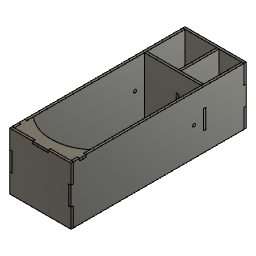
WeldingGearCubby (Autodesk Fusion 360 design; units mm, degrees)
Autodesk Fusion 360 part; units mm, degrees
note: some values were not read from the file. Set by a fixed rule: which face or edge a step refers to.
(part 1 of 2)
sketch "Sketch1" plane through (0, 0, 0) normal (0, 1, 0) x (1, 0, 0)
  line L0 (0, 0) -> (254, 0)
  line L1 (254, 0) -> (254, -304.8)
  line L2 (254, -304.8) -> (0, -304.8)
  line L3 (0, -304.8) -> (0, 0)
  line L4 (254, 0) -> (272.288, 0)
  line L5 (272.288, 0) -> (272.288, -304.8)
  line L6 (272.288, -304.8) -> (254, -304.8)
  line L7 (254, -304.8) -> (254, 0)
  line L8 (272.288, 0) -> (453.263, 0)
  line L9 (453.263, 0) -> (453.263, -304.8)
  line L10 (453.263, -304.8) -> (272.288, -304.8)
  line L11 (272.288, -304.8) -> (272.288, 0)
  line L12 (0, 0) -> (-18.288, 0) construction
  line L13 (-18.288, 0) -> (471.551, 0)
  line L14 (-18.288, 0) -> (0, 0)
  line L15 (0, 0) -> (0, -1364.488)
  line L16 (0, -1364.488) -> (-18.288, -1364.488)
  line L17 (-18.288, -1364.488) -> (-18.288, 0)
  line L18 (471.551, 0) -> (453.263, 0)
  line L19 (453.263, 0) -> (453.263, -1364.488)
  line L20 (453.263, -1364.488) -> (471.551, -1364.488)
  line L21 (471.551, -1364.488) -> (471.551, 0)
  line L22 (-18.288, -1364.488) -> (471.551, -1364.488)
  line L23 (471.551, -1364.488) -> (471.551, -1382.776)
  line L24 (471.551, -1382.776) -> (-18.288, -1382.776)
  line L25 (-18.288, -1382.776) -> (-18.288, -1364.488)
  line L26 (0, -304.8) -> (453.263, -304.8)
  line L27 (453.263, -304.8) -> (453.263, -323.088)
  line L28 (453.263, -323.088) -> (0, -323.088)
  line L29 (0, -323.088) -> (0, -304.8)
  line L30 (-18.288, 0) -> (-18.288, 18.288)
  line L31 (471.551, 0) -> (471.551, 18.288)
  line L32 (-18.288, 18.288) -> (471.551, 18.288)
  dimension "d2" = 254
  dimension "d3" = 304.8
  dimension "d4" = 18.288
  dimension "d5" = 304.8
  dimension "d6" = 180.975
  dimension "d7" = 304.8
  dimension "d8" = 18.288
  dimension "d9" = 489.839
  dimension "d10" = 1364.488
  dimension "d11" = 1364.488
  dimension "d12" = 489.839
  dimension "d13" = 18.288
  dimension "d14" = 453.263
  dimension "d15" = 18.288
  dimension "d30" = 18.288
  dimension "d31" = 18.288
  constraint horizontal L0
  constraint vertical L1
  constraint horizontal L2
  constraint vertical L3
  constraint coincident L0.start L3.end
  constraint horizontal L4
  constraint vertical L5
  constraint horizontal L6
  constraint vertical L7
  constraint horizontal L8
  constraint vertical L9
  constraint horizontal L10
  constraint vertical L11
  constraint perpendicular L3 L12
  constraint horizontal L13
  constraint horizontal L14
  constraint vertical L15
  constraint horizontal L16
  constraint vertical L17
  constraint horizontal L18
  constraint vertical L19
  constraint horizontal L20
  constraint vertical L21
  constraint horizontal L22
  constraint vertical L23
  constraint horizontal L24
  constraint vertical L25
  constraint horizontal L26
  constraint vertical L27
  constraint horizontal L28
  constraint vertical L29
  constraint perpendicular L13 L30
  constraint perpendicular L18 L31
  measures "d2" distance of L0.start L0.end
  measures "d3" distance of L0.start L2.end
  measures "d4" distance of L0.end L4.end
  measures "d5" distance of L0.end L1.end
  measures "d6" distance of L4.end L8.end
  measures "d7" distance of L4.end L5.end
  measures "d8" distance of L0.start L12.end
  measures "d9" distance of L12.end L13.end
  measures "d10" distance of L12.end L16.end
  measures "d11" distance of L13.end L20.end
  measures "d12" distance of L16.end L20.end
  measures "d13" distance of L16.end L24.end
  measures "d14" distance of L2.end L9.end
  measures "d15" distance of L2.end L28.end
  measures "d30" distance of L12.end L30.end
  measures "d31" distance of L13.end L31.end
extrude "Extrude1" add sketch "Sketch1" against normal blind 457.2 contours L0 L4 L8 L13 L14 L18 L30 L31 L32 makes body 1
copy_body "Body->Comp1" bodies 1 removing the originals makes body 2 in component "Top"
extrude "Extrude1'" add sketch "Sketch1" against normal blind 457.2 separate body contours L3 L13 L14 L15 L16 L17 L22 L29 makes body 3 in component "RightSide"
extrude "Extrude1''" add sketch "Sketch1" against normal blind 457.2 separate body contours L9 L13 L18 L19 L20 L21 L22 L27 makes body 4 in component "LeftSide"
extrude "Extrude1'''" add sketch "Sketch1" against normal blind 457.2 separate body contours L1 L4 L5 L6 L7 L11 L13 L26 makes body 5 in component "Divider"
extrude "Extrude1''''" add sketch "Sketch1" against normal blind 457.2 separate body contours L2 L6 L10 L15 L19 L26 L27 L28 L29 makes body 6 in component "Shelf"
extrude "Extrude1'''''" add sketch "Sketch1" against normal blind 457.2 separate body contours L16 L20 L22 L23 L24 L25 makes body 7 in component "Bottom"
extrude "Extrude1''''''" add sketch "Sketch1" along normal blind 18.288 separate body makes body 8 in component "Back"
sketch "Sketch2" plane through (0, 0, -18.288) normal (0, 0, -1) x (-1, 0, 0)
  line L0 (18.288, 0) -> (-471.551, 0)
  line L1 (-471.551, 0) -> (-471.551, -457.2)
  line L2 (-471.551, -457.2) -> (18.288, -457.2)
  line L3 (18.288, -457.2) -> (18.288, 0)
  line L4 (-150.4315, -18.288) -> (-302.8315, -18.288)
  line L5 (-302.8315, -18.288) -> (-302.8315, 18.288)
  line L6 (-302.8315, 18.288) -> (-150.4315, 18.288)
  line L7 (-150.4315, 18.288) -> (-150.4315, -18.288)
  line L8 (-150.4315, -18.288) -> (-302.8315, 18.288) construction
  line L9 (-302.8315, -18.288) -> (-150.4315, 18.288) construction
  line L10 (-453.263, -304.8) -> (-489.839, -304.8)
  line L11 (-489.839, -304.8) -> (-489.839, -152.4)
  line L12 (-489.839, -152.4) -> (-453.263, -152.4)
  line L13 (-453.263, -152.4) -> (-453.263, -304.8)
  line L14 (-453.263, -304.8) -> (-489.839, -152.4) construction
  line L15 (-489.839, -304.8) -> (-453.263, -152.4) construction
  line L16 (36.576, -304.8) -> (0, -304.8)
  line L17 (0, -304.8) -> (0, -152.4)
  line L18 (0, -152.4) -> (36.576, -152.4)
  line L19 (36.576, -152.4) -> (36.576, -304.8)
  line L20 (36.576, -304.8) -> (0, -152.4) construction
  line L21 (0, -304.8) -> (36.576, -152.4) construction
  point P0 (-226.6315, 0)
  point P1 (-471.551, -228.6)
  point P2 (18.288, -228.6)
  dimension "d32" = 152.4
  dimension "d33" = 36.576
  dimension "d34" = 36.576
  dimension "d35" = 152.4
  dimension "d36" = 36.576
  dimension "d37" = 152.4
  constraint horizontal L4
  constraint perpendicular L4 L5
  constraint parallel L4 L6
  constraint parallel L5 L7
  constraint coincident L8 P0
  constraint coincident L9 P0
  constraint midpoint L0 P0
  constraint horizontal L10
  constraint perpendicular L10 L11
  constraint parallel L10 L12
  constraint parallel L11 L13
  constraint coincident L14 P1
  constraint coincident L15 P1
  constraint midpoint L1 P1
  constraint horizontal L16
  constraint perpendicular L16 L17
  constraint parallel L16 L18
  constraint parallel L17 L19
  constraint coincident L20 P2
  constraint coincident L21 P2
  constraint midpoint L3 P2
  measures "d32" distance of L5.end L6.end
  measures "d33" distance of L4.end L5.end
  measures "d34" distance of L11.end L12.end
  measures "d35" distance of L10.end L11.end
  measures "d36" distance of L17.end L18.end
  measures "d37" distance of L16.end L17.end
extrude "Extrude1'''''''" add sketch "Sketch2" against normal up to surface (18.288 mm away) contours L0 L5 L6 L7 bodies 2 in component "Top"
extrude "Extrude2" cut sketch "Sketch2" against normal up to surface (18.288 mm away) contours L3 L16 L17 L18 | L1 L10 L12 L13 bodies 2 in component "Top"
sketch "Sketch3" plane through (0, 0, 1382.776) normal (0, 0, 1) x (1, 0, 0)
  line L0 (471.551, 0) -> (-18.288, 0)
  line L1 (-18.288, 0) -> (-18.288, -457.2)
  line L2 (-18.288, -457.2) -> (471.551, -457.2)
  line L3 (471.551, -457.2) -> (471.551, 0)
  line L4 (489.839, -304.8) -> (453.263, -304.8)
  line L5 (453.263, -304.8) -> (453.263, -152.4)
  line L6 (453.263, -152.4) -> (489.839, -152.4)
  line L7 (489.839, -152.4) -> (489.839, -304.8)
  line L8 (489.839, -304.8) -> (453.263, -152.4) construction
  line L9 (453.263, -304.8) -> (489.839, -152.4) construction
  line L10 (0, -304.8) -> (-36.576, -304.8)
  line L11 (-36.576, -304.8) -> (-36.576, -152.4)
  line L12 (-36.576, -152.4) -> (0, -152.4)
  line L13 (0, -152.4) -> (0, -304.8)
  line L14 (0, -304.8) -> (-36.576, -152.4) construction
  line L15 (-36.576, -304.8) -> (0, -152.4) construction
  line L16 (312.4324, 18.288) -> (140.8306, 18.288)
  line L17 (140.8306, 18.288) -> (140.8306, -18.288)
  line L18 (140.8306, -18.288) -> (312.4324, -18.288)
  line L19 (312.4324, -18.288) -> (312.4324, 18.288)
  line L20 (312.4324, 18.288) -> (140.8306, -18.288) construction
  line L21 (140.8306, 18.288) -> (312.4324, -18.288) construction
  point P0 (471.551, -228.6)
  point P1 (-18.288, -228.6)
  point P2 (226.6315, 0)
  dimension "d42" = 36.576
  dimension "d43" = 152.4
  dimension "d44" = 36.576
  dimension "d45" = 152.4
  dimension "d46" = 36.576
  constraint horizontal L4
  constraint perpendicular L4 L5
  constraint parallel L4 L6
  constraint parallel L5 L7
  constraint coincident L8 P0
  constraint coincident L9 P0
  constraint midpoint L3 P0
  constraint horizontal L10
  constraint perpendicular L10 L11
  constraint parallel L10 L12
  constraint parallel L11 L13
  constraint coincident L14 P1
  constraint coincident L15 P1
  constraint midpoint L1 P1
  constraint horizontal L16
  constraint perpendicular L16 L17
  constraint parallel L16 L18
  constraint parallel L17 L19
  constraint coincident L20 P2
  constraint coincident L21 P2
  constraint midpoint L0 P2
  measures "d42" distance of L5.end L6.end
  measures "d43" distance of L4.end L5.end
  measures "d44" distance of L11.end L12.end
  measures "d45" distance of L10.end L11.end
  measures "d46" distance of L16.end L17.end
extrude "Extrude2'" add sketch "Sketch3" against normal up to surface (18.288 mm away) contours L0 L16 L17 L19 bodies 7 in component "Bottom"
extrude "Extrude3" cut sketch "Sketch3" against normal up to surface (18.288 mm away) contours L3 L4 L5 L6 | L1 L10 L12 L13 bodies 7 in component "Bottom"
sketch "Sketch4" plane through (0, 0, -18.288) normal (0, 0, -1) x (-1, 0, 0)
  line L0 (-453.263, -304.8) -> (-471.551, -304.8)
  line L1 (-471.551, -304.8) -> (-471.551, -457.2)
  line L2 (-471.551, -457.2) -> (18.288, -457.2)
  line L3 (18.288, -457.2) -> (18.288, -304.8)
  line L4 (18.288, -304.8) -> (0, -304.8)
  line L5 (0, -304.8) -> (0, -152.4)
  line L6 (0, -152.4) -> (18.288, -152.4)
  line L7 (18.288, -152.4) -> (18.288, 0)
  line L8 (18.288, 0) -> (-150.4315, 0)
  line L9 (-150.4315, 0) -> (-150.4315, 18.288)
  line L10 (-150.4315, 18.288) -> (-302.8315, 18.288)
  line L11 (-302.8315, 18.288) -> (-302.8315, 0)
  line L12 (-302.8315, 0) -> (-471.551, 0)
  line L13 (-471.551, 0) -> (-471.551, -152.4)
  line L14 (-471.551, -152.4) -> (-453.263, -152.4)
  line L15 (-453.263, -152.4) -> (-453.263, -304.8)
  line L16 (-453.263, -228.6) -> (-263.144, -228.6) construction
  line L17 (-254, -304.8) -> (-272.288, -304.8)
  line L18 (-272.288, -304.8) -> (-272.288, -152.4)
  line L19 (-272.288, -152.4) -> (-254, -152.4)
  line L20 (-254, -152.4) -> (-254, -304.8)
  line L21 (-254, -304.8) -> (-272.288, -152.4) construction
  line L22 (-272.288, -304.8) -> (-254, -152.4) construction
  point P0 (-263.144, -228.6)
  dimension "d51" = 190.119
  dimension "d52" = 18.288
  dimension "d53" = 152.4
  constraint midpoint L15 L16.start
  constraint perpendicular L15 L16
  constraint horizontal L17
  constraint perpendicular L17 L18
  constraint parallel L17 L19
  constraint parallel L18 L20
  constraint coincident L21 P0
  constraint coincident L22 P0
  constraint coincident P0 L16.end
  measures "d51" distance of L16.start P0
  measures "d52" distance of L18.end L19.end
  measures "d53" distance of L17.end L18.end
extrude "Extrude3'" cut sketch "Sketch4" against normal blind 18.288 contours L17 L18 L19 L20 bodies 2 in component "Top"
sketch "Sketch5" plane through (0, 0, 304.8) normal (0, 0, -1) x (-1, 0, 0)
  line L0 (0, 0) -> (-453.263, 0)
  line L1 (-453.263, 0) -> (-453.263, -457.2)
  line L2 (-453.263, -457.2) -> (0, -457.2)
  line L3 (0, -457.2) -> (0, 0)
  line L4 (-150.4315, 18.288) -> (-302.8315, 18.288)
  line L5 (-302.8315, 18.288) -> (-302.8315, -18.288)
  line L6 (-302.8315, -18.288) -> (-150.4315, -18.288)
  line L7 (-150.4315, -18.288) -> (-150.4315, 18.288)
  line L8 (-150.4315, 18.288) -> (-302.8315, -18.288) construction
  line L9 (-302.8315, 18.288) -> (-150.4315, -18.288) construction
  line L10 (18.288, -304.8) -> (-18.288, -304.8)
  line L11 (-18.288, -304.8) -> (-18.288, -152.4)
  line L12 (-18.288, -152.4) -> (18.288, -152.4)
  line L13 (18.288, -152.4) -> (18.288, -304.8)
  line L14 (18.288, -304.8) -> (-18.288, -152.4) construction
  line L15 (-18.288, -304.8) -> (18.288, -152.4) construction
  line L16 (-471.551, -304.8) -> (-434.975, -304.8)
  line L17 (-434.975, -304.8) -> (-434.975, -152.4)
  line L18 (-434.975, -152.4) -> (-471.551, -152.4)
  line L19 (-471.551, -152.4) -> (-471.551, -304.8)
  line L20 (-471.551, -304.8) -> (-434.975, -152.4) construction
  line L21 (-434.975, -304.8) -> (-471.551, -152.4) construction
  point P0 (-226.6315, 0)
  point P1 (0, -228.6)
  point P2 (-453.263, -228.6)
  dimension "d56" = 152.4
  dimension "d57" = 36.576
  dimension "d58" = 36.576
  dimension "d59" = 36.576
  constraint horizontal L4
  constraint perpendicular L4 L5
  constraint parallel L4 L6
  constraint parallel L5 L7
  constraint coincident L8 P0
  constraint coincident L9 P0
  constraint midpoint L0 P0
  constraint horizontal L10
  constraint perpendicular L10 L11
  constraint parallel L10 L12
  constraint parallel L11 L13
  constraint coincident L14 P1
  constraint coincident L15 P1
  constraint midpoint L3 P1
  constraint horizontal L16
  constraint perpendicular L16 L17
  constraint parallel L16 L18
  constraint parallel L17 L19
  constraint coincident L20 P2
  constraint coincident L21 P2
  constraint midpoint L1 P2
  measures "d56" distance of L5.end L6.end
  measures "d57" distance of L4.end L5.end
  measures "d58" distance of L11.end L12.end
  measures "d59" distance of L17.end L18.end
extrude "Extrude2''" add sketch "Sketch5" against normal up to surface (18.288 mm away) contours L0 L4 L5 L7 | L3 L10 L12 L13 | L1 L16 L18 L19 bodies 6 in component "Shelf"
sketch "Sketch6" plane through (0, 0, 304.8) normal (0, 0, -1) x (-1, 0, 0)
  line L0 (0, 0) -> (-150.4315, 0)
  line L1 (-150.4315, 0) -> (-150.4315, 18.288)
  line L2 (-150.4315, 18.288) -> (-302.8315, 18.288)
  line L3 (-302.8315, 18.288) -> (-302.8315, 0)
  line L4 (-302.8315, 0) -> (-453.263, 0)
  line L5 (-453.263, 0) -> (-453.263, -152.4)
  line L6 (-453.263, -152.4) -> (-471.551, -152.4)
  line L7 (-471.551, -152.4) -> (-471.551, -304.8)
  line L8 (-471.551, -304.8) -> (-453.263, -304.8)
  line L9 (-453.263, -304.8) -> (-453.263, -457.2)
  line L10 (-453.263, -457.2) -> (0, -457.2)
  line L11 (0, -457.2) -> (0, -304.8)
  line L12 (0, -304.8) -> (18.288, -304.8)
  line L13 (18.288, -304.8) -> (18.288, -152.4)
  line L14 (18.288, -152.4) -> (0, -152.4)
  line L15 (0, -152.4) -> (0, 0)
  line L16 (-471.551, -228.6) -> (-263.144, -228.6) construction
  line L17 (-254, -304.8) -> (-272.288, -304.8)
  line L18 (-272.288, -304.8) -> (-272.288, -152.4)
  line L19 (-272.288, -152.4) -> (-254, -152.4)
  line L20 (-254, -152.4) -> (-254, -304.8)
  line L21 (-254, -304.8) -> (-272.288, -152.4) construction
  line L22 (-272.288, -304.8) -> (-254, -152.4) construction
  point P0 (-263.144, -228.6)
  dimension "d62" = 208.407
  dimension "d63" = 18.288
  dimension "d64" = 152.4
  constraint midpoint L7 L16.start
  constraint perpendicular L7 L16
  constraint horizontal L17
  constraint perpendicular L17 L18
  constraint parallel L17 L19
  constraint parallel L18 L20
  constraint coincident L21 P0
  constraint coincident L22 P0
  constraint coincident P0 L16.end
  measures "d62" distance of L16.start P0
  measures "d63" distance of L18.end L19.end
  measures "d64" distance of L17.end L18.end
extrude "Extrude3''" cut sketch "Sketch6" against normal up to surface (18.288 mm away) contours L17 L18 L19 L20 bodies 6 in component "Shelf"
sketch "Sketch7" plane through (471.551, 0, 0) normal (1, 0, 0) x (0, 0, -1)
  line L0 (0, 0) -> (-1364.488, 0)
  line L1 (-1364.488, 0) -> (-1364.488, -457.2)
  line L2 (-1364.488, -457.2) -> (0, -457.2)
  line L3 (0, -457.2) -> (0, 0)
  line L4 (18.288, -304.8) -> (-18.288, -304.8)
  line L5 (-18.288, -304.8) -> (-18.288, -152.4)
  line L6 (-18.288, -152.4) -> (18.288, -152.4)
  line L7 (18.288, -152.4) -> (18.288, -304.8)
  line L8 (18.288, -304.8) -> (-18.288, -152.4) construction
  line L9 (-18.288, -304.8) -> (18.288, -152.4) construction
  line L10 (0, -228.6) -> (-313.944, -228.6) construction
  line L11 (-304.8, -304.8) -> (-323.088, -304.8)
  line L12 (-323.088, -304.8) -> (-323.088, -152.4)
  line L13 (-323.088, -152.4) -> (-304.8, -152.4)
  line L14 (-304.8, -152.4) -> (-304.8, -304.8)
  line L15 (-304.8, -304.8) -> (-323.088, -152.4) construction
  line L16 (-323.088, -304.8) -> (-304.8, -152.4) construction
  line L17 (-1382.776, -304.8) -> (-1346.2, -304.8)
  line L18 (-1346.2, -304.8) -> (-1346.2, -152.4)
  line L19 (-1346.2, -152.4) -> (-1382.776, -152.4)
  line L20 (-1382.776, -152.4) -> (-1382.776, -304.8)
  line L21 (-1382.776, -304.8) -> (-1346.2, -152.4) construction
  line L22 (-1346.2, -304.8) -> (-1382.776, -152.4) construction
  point P0 (0, -228.6)
  point P1 (-313.944, -228.6)
  point P2 (-1364.488, -228.6)
  dimension "d67" = 36.576
  dimension "d68" = 313.944
  dimension "d69" = 18.288
  dimension "d70" = 152.4
  dimension "d71" = 36.576
  dimension "d72" = 152.4
  constraint horizontal L4
  constraint perpendicular L4 L5
  constraint parallel L4 L6
  constraint parallel L5 L7
  constraint coincident L8 P0
  constraint coincident L9 P0
  constraint midpoint L3 P0
  constraint coincident P0 L10.start
  constraint perpendicular L5 L10
  constraint horizontal L11
  constraint perpendicular L11 L12
  constraint parallel L11 L13
  constraint parallel L12 L14
  constraint coincident L15 P1
  constraint coincident L16 P1
  constraint coincident P1 L10.end
  constraint horizontal L17
  constraint perpendicular L17 L18
  constraint parallel L17 L19
  constraint parallel L18 L20
  constraint coincident L21 P2
  constraint coincident L22 P2
  constraint midpoint L1 P2
  measures "d67" distance of L5.end L6.end
  measures "d68" distance of P0 P1
  measures "d69" distance of L12.end L13.end
  measures "d70" distance of L11.end L12.end
  measures "d71" distance of L18.end L19.end
  measures "d72" distance of L17.end L18.end
extrude "Extrude2'''" add sketch "Sketch7" against normal up to surface (18.288 mm away) contours L3 L4 L6 L7 | L1 L17 L19 L20 bodies 4 in component "LeftSide"
extrude "Extrude3'''" cut sketch "Sketch7" against normal up to surface (18.288 mm away) contours L11 L12 L13 L14 bodies 4 in component "LeftSide"
sketch "Sketch8" plane through (-18.288, 0, 0) normal (-1, 0, 0) x (0, 0, 1)
  line L0 (1364.488, 0) -> (0, 0)
  line L1 (0, 0) -> (0, -457.2)
  line L2 (0, -457.2) -> (1364.488, -457.2)
  line L3 (1364.488, -457.2) -> (1364.488, 0)
  line L4 (18.288, -304.8) -> (-18.288, -304.8)
  line L5 (-18.288, -304.8) -> (-18.288, -152.4)
  line L6 (-18.288, -152.4) -> (18.288, -152.4)
  line L7 (18.288, -152.4) -> (18.288, -304.8)
  line L8 (18.288, -304.8) -> (-18.288, -152.4) construction
  line L9 (-18.288, -304.8) -> (18.288, -152.4) construction
  line L10 (1382.776, -304.8) -> (1346.2, -304.8)
  line L11 (1346.2, -304.8) -> (1346.2, -152.4)
  line L12 (1346.2, -152.4) -> (1382.776, -152.4)
  line L13 (1382.776, -152.4) -> (1382.776, -304.8)
  line L14 (1382.776, -304.8) -> (1346.2, -152.4) construction
  line L15 (1346.2, -304.8) -> (1382.776, -152.4) construction
  line L16 (0, -228.6) -> (313.944, -228.6) construction
  line L17 (323.088, -304.8) -> (304.8, -304.8)
  line L18 (304.8, -304.8) -> (304.8, -152.4)
  line L19 (304.8, -152.4) -> (323.088, -152.4)
  line L20 (323.088, -152.4) -> (323.088, -304.8)
  line L21 (323.088, -304.8) -> (304.8, -152.4) construction
  line L22 (304.8, -304.8) -> (323.088, -152.4) construction
  point P0 (0, -228.6)
  point P1 (1364.488, -228.6)
  point P2 (313.944, -228.6)
  dimension "d77" = 36.576
  dimension "d78" = 152.4
  dimension "d79" = 36.576
  dimension "d80" = 152.4
  dimension "d81" = 313.944
  dimension "d82" = 18.288
  dimension "d83" = 152.4
  constraint horizontal L4
  constraint perpendicular L4 L5
  constraint parallel L4 L6
  constraint parallel L5 L7
  constraint coincident L8 P0
  constraint coincident L9 P0
  constraint midpoint L1 P0
  constraint horizontal L10
  constraint perpendicular L10 L11
  constraint parallel L10 L12
  constraint parallel L11 L13
  constraint coincident L14 P1
  constraint coincident L15 P1
  constraint midpoint L3 P1
  constraint coincident P0 L16.start
  constraint perpendicular L7 L16
  constraint horizontal L17
  constraint perpendicular L17 L18
  constraint parallel L17 L19
  constraint parallel L18 L20
  constraint coincident L21 P2
  constraint coincident L22 P2
  constraint coincident P2 L16.end
  measures "d77" distance of L5.end L6.end
  measures "d78" distance of L4.end L5.end
  measures "d79" distance of L11.end L12.end
  measures "d80" distance of L10.end L11.end
  measures "d81" distance of P0 P2
  measures "d82" distance of L18.end L19.end
  measures "d83" distance of L17.end L18.end
extrude "Extrude2''''" add sketch "Sketch8" against normal up to surface (18.288 mm away) contours L3 L10 L12 L13 | L1 L4 L5 L6 bodies 3 in component "RightSide"
extrude "Extrude3''''" cut sketch "Sketch8" against normal up to surface (18.288 mm away) contours L17 L18 L19 L20 bodies 3 in component "RightSide"
sketch "Sketch9" plane through (272.288, 0, 0) normal (1, 0, 0) x (0, 0, -1)
  line L0 (0, 0) -> (-304.8, 0)
  line L1 (-304.8, 0) -> (-304.8, -457.2)
  line L2 (-304.8, -457.2) -> (0, -457.2)
  line L3 (0, -457.2) -> (0, 0)
  line L4 (18.288, -304.8) -> (-18.288, -304.8)
  line L5 (-18.288, -304.8) -> (-18.288, -152.4)
  line L6 (-18.288, -152.4) -> (18.288, -152.4)
  line L7 (18.288, -152.4) -> (18.288, -304.8)
  line L8 (18.288, -304.8) -> (-18.288, -152.4) construction
  line L9 (-18.288, -304.8) -> (18.288, -152.4) construction
  line L10 (-286.512, -304.8) -> (-323.088, -304.8)
  line L11 (-323.088, -304.8) -> (-323.088, -152.4)
  line L12 (-323.088, -152.4) -> (-286.512, -152.4)
  line L13 (-286.512, -152.4) -> (-286.512, -304.8)
  line L14 (-286.512, -304.8) -> (-323.088, -152.4) construction
  line L15 (-323.088, -304.8) -> (-286.512, -152.4) construction
  point P0 (0, -228.6)
  point P1 (-304.8, -228.6)
  dimension "d88" = 36.576
  dimension "d89" = 152.4
  dimension "d90" = 36.576
  constraint horizontal L4
  constraint perpendicular L4 L5
  constraint parallel L4 L6
  constraint parallel L5 L7
  constraint coincident L8 P0
  constraint coincident L9 P0
  constraint midpoint L3 P0
  constraint horizontal L10
  constraint perpendicular L10 L11
  constraint parallel L10 L12
  constraint parallel L11 L13
  constraint coincident L14 P1
  constraint coincident L15 P1
  constraint midpoint L1 P1
  measures "d88" distance of L5.end L6.end
  measures "d89" distance of L4.end L5.end
  measures "d90" distance of L11.end L12.end
extrude "Extrude2'''''" add sketch "Sketch9" against normal up to surface (18.288 mm away) contours L3 L4 L6 L7 | L1 L10 L11 L12 bodies 5 in component "Divider"
sketch "Sketch10" plane through (0, 18.288, 0) normal (0, 1, 0) x (-1, 0, 0)
  line L0 (18.288, -18.288) -> (18.288, 1382.776)
  line L1 (18.288, 1382.776) -> (-471.551, 1382.776)
  line L2 (-471.551, 1382.776) -> (-471.551, -18.288)
  line L3 (-471.551, -18.288) -> (18.288, -18.288)
  line L4 (-226.6315, -18.288) -> (-226.6315, 313.944) construction
  line L5 (-302.8315, 323.088) -> (-150.4315, 323.088)
  line L6 (-150.4315, 323.088) -> (-150.4315, 304.8)
  line L7 (-150.4315, 304.8) -> (-302.8315, 304.8)
  line L8 (-302.8315, 304.8) -> (-302.8315, 323.088)
  line L9 (-302.8315, 323.088) -> (-150.4315, 304.8) construction
  line L10 (-150.4315, 323.088) -> (-302.8315, 304.8) construction
  line L11 (-302.8315, 0) -> (-150.4315, 0)
  line L12 (-150.4315, 0) -> (-150.4315, -36.576)
  line L13 (-150.4315, -36.576) -> (-302.8315, -36.576)
  line L14 (-302.8315, -36.576) -> (-302.8315, 0)
  line L15 (-302.8315, 0) -> (-150.4315, -36.576) construction
  line L16 (-150.4315, 0) -> (-302.8315, -36.576) construction
  line L17 (-302.8315, 1401.064) -> (-150.4315, 1401.064)
  line L18 (-150.4315, 1401.064) -> (-150.4315, 1364.488)
  line L19 (-150.4315, 1364.488) -> (-302.8315, 1364.488)
  line L20 (-302.8315, 1364.488) -> (-302.8315, 1401.064)
  line L21 (-302.8315, 1401.064) -> (-150.4315, 1364.488) construction
  line L22 (-150.4315, 1401.064) -> (-302.8315, 1364.488) construction
  line L23 (-489.839, 758.444) -> (-453.263, 758.444)
  line L24 (-453.263, 758.444) -> (-453.263, 606.044)
  line L25 (-453.263, 606.044) -> (-489.839, 606.044)
  line L26 (-489.839, 606.044) -> (-489.839, 758.444)
  line L27 (-489.839, 758.444) -> (-453.263, 606.044) construction
  line L28 (-453.263, 758.444) -> (-489.839, 606.044) construction
  line L29 (0, 758.444) -> (36.576, 758.444)
  line L30 (36.576, 758.444) -> (36.576, 606.044)
  line L31 (36.576, 606.044) -> (0, 606.044)
  line L32 (0, 606.044) -> (0, 758.444)
  line L33 (0, 758.444) -> (36.576, 606.044) construction
  line L34 (36.576, 758.444) -> (0, 606.044) construction
  point P0 (-226.6315, 313.944)
  point P1 (-226.6315, -18.288)
  point P2 (-226.6315, 1382.776)
  point P3 (-471.551, 682.244)
  point P4 (18.288, 682.244)
  dimension "d93" = 332.232
  dimension "d94" = 152.4
  dimension "d95" = 18.288
  dimension "d96" = 152.4
  dimension "d97" = 36.576
  dimension "d98" = 152.4
  dimension "d99" = 36.576
  dimension "d100" = 36.576
  dimension "d101" = 152.4
  dimension "d102" = 36.576
  dimension "d103" = 152.4
  constraint midpoint L3 P1
  constraint perpendicular L3 L4
  constraint horizontal L5
  constraint perpendicular L5 L6
  constraint parallel L5 L7
  constraint parallel L6 L8
  constraint coincident L9 P0
  constraint coincident L10 P0
  constraint coincident P0 L4.end
  constraint horizontal L11
  constraint perpendicular L11 L12
  constraint parallel L11 L13
  constraint parallel L12 L14
  constraint coincident L15 P1
  constraint coincident L16 P1
  constraint coincident P1 L4.start
  constraint horizontal L17
  constraint perpendicular L17 L18
  constraint parallel L17 L19
  constraint parallel L18 L20
  constraint coincident L21 P2
  constraint coincident L22 P2
  constraint midpoint L1 P2
  constraint horizontal L23
  constraint perpendicular L23 L24
  constraint parallel L23 L25
  constraint parallel L24 L26
  constraint coincident L27 P3
  constraint coincident L28 P3
  constraint midpoint L2 P3
  constraint horizontal L29
  constraint perpendicular L29 L30
  constraint parallel L29 L31
  constraint parallel L30 L32
  constraint coincident L33 P4
  constraint coincident L34 P4
  constraint midpoint L0 P4
  measures "d93" distance of P1 P0
  measures "d94" distance of L6.end L7.end
  measures "d95" distance of L5.end L6.end
  measures "d96" distance of L12.end L13.end
  measures "d97" distance of L11.end L12.end
  measures "d98" distance of L18.end L19.end
  measures "d99" distance of L17.end L18.end
  measures "d100" distance of L24.end L25.end
  measures "d101" distance of L23.end L24.end
  measures "d102" distance of L30.end L31.end
  measures "d103" distance of L29.end L30.end
extrude "Extrude2''''''" cut sketch "Sketch10" against normal up to surface (18.288 mm away) contours L0 L29 L31 L32 | L3 L11 L12 L14 | L1 L18 L19 L20 | L2 L23 L24 L25 | L5 L6 L7 L8 bodies 8 in component "Back"
sketch "Sketch11" plane through (471.551, 0, 0) normal (1, 0, 0) x (0, 0, -1)
  line L0 (-304.8, -152.4) -> (-304.8, -304.8)
  line L1 (-304.8, -304.8) -> (-323.088, -304.8)
  line L2 (-323.088, -304.8) -> (-323.088, -152.4)
  line L3 (-323.088, -152.4) -> (-304.8, -152.4)
  line L4 (0, 0) -> (-1364.488, 0)
  line L5 (-1364.488, 0) -> (-1364.488, -152.4)
  line L6 (-1364.488, -152.4) -> (-1382.776, -152.4)
  line L7 (-1382.776, -152.4) -> (-1382.776, -304.8)
  line L8 (-1382.776, -304.8) -> (-1364.488, -304.8)
  line L9 (-1364.488, -304.8) -> (-1364.488, -457.2)
  line L10 (-1364.488, -457.2) -> (0, -457.2)
  line L11 (0, -457.2) -> (0, -304.8)
  line L12 (0, -304.8) -> (18.288, -304.8)
  line L13 (18.288, -304.8) -> (18.288, -152.4)
  line L14 (18.288, -152.4) -> (0, -152.4)
  line L15 (0, -152.4) -> (0, 0)
  line L16 (-606.044, 18.288) -> (-758.444, 18.288)
  line L17 (-758.444, 18.288) -> (-758.444, -18.288)
  line L18 (-758.444, -18.288) -> (-606.044, -18.288)
  line L19 (-606.044, -18.288) -> (-606.044, 18.288)
  line L20 (-606.044, 18.288) -> (-758.444, -18.288) construction
  line L21 (-758.444, 18.288) -> (-606.044, -18.288) construction
  point P0 (-682.244, 0)
  dimension "d106" = 152.4
  dimension "d107" = 36.576
  constraint horizontal L16
  constraint perpendicular L16 L17
  constraint parallel L16 L18
  constraint parallel L17 L19
  constraint coincident L20 P0
  constraint coincident L21 P0
  constraint midpoint L4 P0
  measures "d106" distance of L17.end L18.end
  measures "d107" distance of L16.end L17.end
extrude "Extrude4" add sketch "Sketch11" against normal up to surface (18.288 mm away) contours L4 L16 L17 L19 bodies 4 in component "LeftSide"
sketch "Sketch12" plane through (-18.288, 0, 0) normal (-1, 0, 0) x (0, 0, 1)
  line L0 (323.088, -152.4) -> (323.088, -304.8)
  line L1 (323.088, -304.8) -> (304.8, -304.8)
  line L2 (304.8, -304.8) -> (304.8, -152.4)
  line L3 (304.8, -152.4) -> (323.088, -152.4)
  line L4 (1364.488, 0) -> (0, 0)
  line L5 (0, 0) -> (0, -152.4)
  line L6 (0, -152.4) -> (-18.288, -152.4)
  line L7 (-18.288, -152.4) -> (-18.288, -304.8)
  line L8 (-18.288, -304.8) -> (0, -304.8)
  line L9 (0, -304.8) -> (0, -457.2)
  line L10 (0, -457.2) -> (1364.488, -457.2)
  line L11 (1364.488, -457.2) -> (1364.488, -304.8)
  line L12 (1364.488, -304.8) -> (1382.776, -304.8)
  line L13 (1382.776, -304.8) -> (1382.776, -152.4)
  line L14 (1382.776, -152.4) -> (1364.488, -152.4)
  line L15 (1364.488, -152.4) -> (1364.488, 0)
  line L16 (758.444, 18.288) -> (606.044, 18.288)
  line L17 (606.044, 18.288) -> (606.044, -18.288)
  line L18 (606.044, -18.288) -> (758.444, -18.288)
  line L19 (758.444, -18.288) -> (758.444, 18.288)
  line L20 (758.444, 18.288) -> (606.044, -18.288) construction
  line L21 (606.044, 18.288) -> (758.444, -18.288) construction
  point P0 (682.244, 0)
  dimension "d110" = 152.4
  dimension "d111" = 36.576
  constraint horizontal L16
  constraint perpendicular L16 L17
  constraint parallel L16 L18
  constraint parallel L17 L19
  constraint coincident L20 P0
  constraint coincident L21 P0
  constraint midpoint L4 P0
  measures "d110" distance of L17.end L18.end
  measures "d111" distance of L16.end L17.end
extrude "Extrude4'" add sketch "Sketch12" against normal up to surface (18.288 mm away) contours L4 L16 L17 L19 bodies 3 in component "RightSide"
sketch "Sketch13" plane through (471.551, 0, 0) normal (1, 0, 0) x (0, 0, -1)
  line L0 (-304.8, -152.4) -> (-304.8, -304.8)
  line L1 (-304.8, -304.8) -> (-323.088, -304.8)
  line L2 (-323.088, -304.8) -> (-323.088, -152.4)
  line L3 (-323.088, -152.4) -> (-304.8, -152.4)
  line L4 (-758.444, 0) -> (-1364.488, 0)
  line L5 (-1364.488, 0) -> (-1364.488, -152.4)
  line L6 (-1364.488, -152.4) -> (-1382.776, -152.4)
  line L7 (-1382.776, -152.4) -> (-1382.776, -304.8)
  line L8 (-1382.776, -304.8) -> (-1364.488, -304.8)
  line L9 (-1364.488, -304.8) -> (-1364.488, -457.2)
  line L10 (-1364.488, -457.2) -> (0, -457.2)
  line L11 (0, -457.2) -> (0, -304.8)
  line L12 (0, -304.8) -> (18.288, -304.8)
  line L13 (18.288, -304.8) -> (18.288, -152.4)
  line L14 (18.288, -152.4) -> (0, -152.4)
  line L15 (0, -152.4) -> (0, 0)
  line L16 (0, 0) -> (-606.044, 0)
  line L17 (-606.044, 0) -> (-606.044, 18.288)
  line L18 (-606.044, 18.288) -> (-758.444, 18.288)
  line L19 (-758.444, 18.288) -> (-758.444, 0)
  line L20 (-323.088, -228.6) -> (-399.288, -228.6) construction
  circle A0 centre (-399.288, -228.6) radius 11.7475
  dimension "d114" = 76.2
  dimension "d115" = 23.495
  constraint midpoint L2 L20.start
  constraint perpendicular L2 L20
  constraint coincident L20.end A0.centre
  measures "d114" distance of L20.start L20.end
  measures "d115" diameter of A0
extrude "Extrude5" cut sketch "Sketch13" against normal up to surface (489.839 mm away) contours A0 bodies 3 in component "RightSide"
extrude "Extrude5'" cut sketch "Sketch13" against normal up to surface (489.839 mm away) contours A0 bodies 4 in component "LeftSide"
move_face "OffsetFaces1" offset -18.288 1 faces at (252.0315, 18.288, 316.992) on bodies 6 in component "Shelf"
move_face "OffsetFaces1'" offset -18.288 1 faces at (255.2318, 18.288, 1370.584) on bodies 7 in component "Bottom"
move_face "OffsetFaces1''" offset -18.288 1 faces at (252.0315, 18.288, -6.096) on bodies 2 in component "Top"
move_face "OffsetFaces1'''" offset -18.288 1 faces at (459.359, 18.288, 656.844) on bodies 4 in component "LeftSide"
move_face "OffsetFaces1''''" offset -18.288 1 faces at (-12.192, 18.288, 707.644) on bodies 3 in component "RightSide"
sketch "Sketch14" plane through (0, 0, 0) normal (0, 1, 0) x (-1, 0, 0)
  line L0 (18.288, 1382.776) -> (-471.551, 1382.776)
  line L1 (-471.551, 1382.776) -> (-471.551, 1364.488)
  line L2 (18.288, 1364.488) -> (18.288, 1382.776)
  line L3 (18.288, 1364.488) -> (0, 1364.488) construction
  line L4 (-471.551, 1364.488) -> (-453.263, 1364.488) construction
  line L5 (0, 1364.488) -> (-165.1, 1364.488)
  line L6 (-453.263, 1364.488) -> (-288.163, 1364.488)
  line L7 (-165.1, 1364.488) -> (-165.1, 1382.776)
  line L8 (-288.163, 1364.488) -> (-288.163, 1382.776)
  line L9 (-165.1, 1382.776) -> (-288.163, 1382.776)
  line L10 (0, 1364.488) -> (0, 1313.688)
  line L11 (0, 1313.688) -> (18.288, 1313.688)
  line L12 (18.288, 1313.688) -> (18.288, 1262.888)
  line L13 (18.288, 1262.888) -> (0, 1262.888)
  line L14 (0, 1262.888) -> (0, 1212.088)
  line L15 (-453.263, 1364.488) -> (-453.263, 1313.688)
  line L16 (-453.263, 1313.688) -> (-471.551, 1313.688)
  line L17 (-471.551, 1313.688) -> (-471.551, 1262.888)
  line L18 (-471.551, 1262.888) -> (-453.263, 1262.888)
  line L19 (-453.263, 1262.888) -> (-453.263, 1212.088)
  arc A0 (0, 1212.088) -> (-453.263, 1212.088) centre (-226.6315, 945.5172) ccw
  dimension "d125" = 18.288
  dimension "d126" = 165.1
  dimension "d127" = 165.1
  dimension "d128" = 50.8
  dimension "d129" = 18.288
  dimension "d130" = 50.8
  dimension "d131" = 50.8
  dimension "d132" = 50.8
  dimension "d133" = 18.288
  dimension "d134" = 50.8
  dimension "d135" = 18.288
  dimension "d136" = 50.8
  constraint coincident L2.start L3.start
  constraint perpendicular L2 L3
  constraint coincident L1.end L4.start
  constraint perpendicular L1 L4
  constraint perpendicular L1 L6
  constraint coincident L0 L7.end
  constraint perpendicular L0 L7
  constraint coincident L0 L8.end
  constraint perpendicular L0 L8
  constraint perpendicular L5 L10
  constraint perpendicular L10 L11
  constraint perpendicular L11 L12
  constraint perpendicular L12 L13
  constraint perpendicular L13 L14
  constraint perpendicular L4 L15
  constraint perpendicular L15 L16
  constraint perpendicular L16 L17
  constraint perpendicular L17 L18
  constraint perpendicular L18 L19
  measures "d125" distance of L1.end L4.end
  measures "d126" distance of L3.end L5.end
  measures "d127" distance of L4.end L6.end
  measures "d128" distance of L3.end L10.end
  measures "d129" distance of L10.end L11.end
  measures "d130" distance of L11.end L12.end
  measures "d131" distance of L13.end L14.end
  measures "d132" distance of L4.end L15.end
  measures "d133" distance of L15.end L16.end
  measures "d134" distance of L16.end L17.end
  measures "d135" distance of L17.end L18.end
  measures "d136" distance of L18.end L19.end
extrude "Extrude1''''''''" add sketch "Sketch14" against normal blind 18.288 separate body makes body 9 in component "BackSupport"
extrude "Extrude6" cut sketch "Sketch14" against normal blind 18.288 bodies 3 in component "RightSide"
extrude "Extrude6'" cut sketch "Sketch14" against normal blind 18.288 bodies 4 in component "LeftSide"
extrude "Extrude4''" cut sketch "Sketch14" against normal blind 18.288 bodies 7 in component "Bottom"
ref_plane "WorkPlane1" through (272.288, -304.8, -18.288) normal (0, 0, 1) x (1, 0, 0)
sketch "Sketch15" plane through (272.288, -304.8, -18.288) normal (0, 0, 1) x (1, 0, 0)
  line L0 (-18.288, 0) -> (0, 0) construction
  line L1 (0, 0) -> (0, 152.4) construction
  line L2 (0, 0) -> (-2.2451, 2.2451) construction
  circle A0 centre (-2.2451, 2.2451) radius 3.175
  dimension "d146" = 3.175
  constraint coincident L0.end L1.start
  constraint coincident L0.end A0
  measures "d146" distance of L0.end L2.end
sweep "Sweep1" cut kept parallel profiles "Sketch15" along 1 edges at (272.288, -304.8, -9.144) section 1 on bodies 2 bodies 2 in component "Top"
ref_plane "WorkPlane2" through (254, -304.8, -18.288) normal (0, 0, 1) x (1, 0, 0)
sketch "Sketch16" plane through (254, -304.8, -18.288) normal (0, 0, 1) x (1, 0, 0)
  line L0 (0, 152.4) -> (0, 0) construction
  line L1 (0, 0) -> (13.7979, 0) construction
  line L2 (0, 0) -> (2.2451, 2.2451) construction
  circle A0 centre (2.2451, 2.2451) radius 3.175
  dimension "d154" = 3.175
  constraint coincident L0.end L1.start
  constraint coincident L0.end A0
  measures "d154" distance of L0.end L2.end
sweep "Sweep2" cut kept parallel profiles "Sketch16" along 1 edges at (254, -304.8, -9.144) section 1 on bodies 2 bodies 2 in component "Top"
ref_plane "WorkPlane3" through (453.263, -304.8, -18.288) normal (0, 0, 1) x (1, 0, 0)
sketch "Sketch17" plane through (453.263, -304.8, -18.288) normal (0, 0, 1) x (1, 0, 0)
  line L0 (0, 0) -> (0, 152.4) construction
  line L1 (18.288, 0) -> (0, 0) construction
  line L2 (0, 0) -> (2.2451, 2.2451) construction
  circle A0 centre (2.2451, 2.2451) radius 3.175
  dimension "d162" = 3.175
  constraint coincident L0.start L1.end
  constraint coincident L0.start A0
  measures "d162" distance of L0.start L2.end
sweep "Sweep3" cut kept parallel profiles "Sketch17" along 1 edges at (453.263, -304.8, -9.144) section 1 on bodies 2 bodies 2 in component "Top"
ref_plane "WorkPlane4" through (0, -304.8, -18.288) normal (0, 0, 1) x (1, 0, 0)
sketch "Sketch18" plane through (0, -304.8, -18.288) normal (0, 0, 1) x (1, 0, 0)
  line L0 (0, 0) -> (-18.288, 0) construction
  line L1 (0, 152.4) -> (0, 0) construction
  line L2 (0, 0) -> (-2.2451, 2.2451) construction
  circle A0 centre (-2.2451, 2.2451) radius 3.175
  dimension "d170" = 3.175
  constraint coincident L0.start L1.end
  constraint coincident L0.start A0
  measures "d170" distance of L0.start L2.end
sweep "Sweep4" cut kept parallel profiles "Sketch18" along 1 edges at (0, -304.8, -9.144) section 1 on bodies 2 bodies 2 in component "Top"
ref_plane "WorkPlane5" through (272.288, -152.4, -18.288) normal (0, 0, 1) x (1, 0, 0)
sketch "Sketch19" plane through (272.288, -152.4, -18.288) normal (0, 0, 1) x (1, 0, 0)
  line L0 (0, 0) -> (-18.288, 0) construction
  line L1 (0, -147.9099) -> (0, 0) construction
  line L2 (0, 0) -> (-2.2451, -2.2451) construction
  circle A0 centre (-2.2451, -2.2451) radius 3.175
  dimension "d178" = 3.175
  constraint coincident L0.start L1.end
  constraint coincident L0.start A0
  measures "d178" distance of L0.start L2.end
sweep "Sweep5" cut kept parallel profiles "Sketch19" along 1 edges at (272.288, -152.4, -9.144) section 1 on bodies 2 bodies 2 in component "Top"
ref_plane "WorkPlane6" through (0, -152.4, -18.288) normal (0, 0, 1) x (1, 0, 0)
sketch "Sketch20" plane through (0, -152.4, -18.288) normal (0, 0, 1) x (1, 0, 0)
  line L0 (0, 0) -> (0, -147.9099) construction
  line L1 (-18.288, 0) -> (0, 0) construction
  line L2 (0, 0) -> (-2.2451, -2.2451) construction
  circle A0 centre (-2.2451, -2.2451) radius 3.175
  dimension "d186" = 3.175
  constraint coincident L0.start L1.end
  constraint coincident L0.start A0
  measures "d186" distance of L0.start L2.end
sweep "Sweep6" cut kept parallel profiles "Sketch20" along 1 edges at (0, -152.4, -9.144) section 1 on bodies 2 bodies 2 in component "Top"
ref_plane "WorkPlane7" through (254, -152.4, -18.288) normal (0, 0, 1) x (1, 0, 0)
sketch "Sketch21" plane through (254, -152.4, -18.288) normal (0, 0, 1) x (1, 0, 0)
  line L0 (0, 0) -> (13.7979, 0) construction
  line L1 (0, -147.9099) -> (0, 0) construction
  line L2 (0, 0) -> (2.2451, -2.2451) construction
  circle A0 centre (2.2451, -2.2451) radius 3.175
  dimension "d194" = 3.175
  constraint coincident L0.start L1.end
  constraint coincident L0.start A0
  measures "d194" distance of L0.start L2.end
sweep "Sweep7" cut kept parallel profiles "Sketch21" along 1 edges at (254, -152.4, -9.144) section 1 on bodies 2 bodies 2 in component "Top"
ref_plane "WorkPlane8" through (453.263, -152.4, -18.288) normal (0, 0, 1) x (1, 0, 0)
sketch "Sketch22" plane through (453.263, -152.4, -18.288) normal (0, 0, 1) x (1, 0, 0)
  line L0 (0, 0) -> (18.288, 0) construction
  line L1 (0, -147.9099) -> (0, 0) construction
  line L2 (0, 0) -> (2.2451, -2.2451) construction
  circle A0 centre (2.2451, -2.2451) radius 3.175
  dimension "d202" = 3.175
  constraint coincident L0.start L1.end
  constraint coincident L0.start A0
  measures "d202" distance of L0.start L2.end
sweep "Sweep8" cut kept parallel profiles "Sketch22" along 1 edges at (453.263, -152.4, -9.144) section 1 on bodies 2 bodies 2 in component "Top"
ref_plane "WorkPlane9" through (-18.288, -304.8, 0) normal (1, 0, 0) x (0, 1, 0)
sketch "Sketch23" plane through (-18.288, -304.8, 0) normal (1, 0, 0) x (0, 1, 0)
  line L0 (0, 0) -> (-152.4, 0) construction
  line L1 (0, -18.288) -> (0, 0) construction
  line L2 (0, 0) -> (-2.2451, -2.2451) construction
  circle A0 centre (-2.2451, -2.2451) radius 3.175
  dimension "d210" = 3.175
  constraint coincident L0.start L1.end
  constraint coincident L0.start A0
  measures "d210" distance of L0.start L2.end
sweep "Sweep1'" cut kept parallel profiles "Sketch23" along 1 edges at (-9.144, -304.8, 0) section 1 on bodies 3 bodies 3 in component "RightSide"
ref_plane "WorkPlane10" through (0, -152.4, 0) normal (-1, 0, 0) x (0, -1, 0)
sketch "Sketch24" plane through (0, -152.4, 0) normal (-1, 0, 0) x (0, -1, 0)
  line L0 (-152.4, 0) -> (0, 0) construction
  line L1 (0, -18.288) -> (0, 0) construction
  line L2 (0, 0) -> (-2.2451, -2.2451) construction
  circle A0 centre (-2.2451, -2.2451) radius 3.175
  dimension "d218" = 3.175
  constraint coincident L0.end L1.end
  constraint coincident L0.end A0
  measures "d218" distance of L0.end L2.end
sweep "Sweep2'" cut kept parallel profiles "Sketch24" along 1 edges at (-9.144, -152.4, 0) section 1 on bodies 3 bodies 3 in component "RightSide"
ref_plane "WorkPlane11" through (-18.288, -304.8, 323.088) normal (1, 0, 0) x (0, 1, 0)
sketch "Sketch25" plane through (-18.288, -304.8, 323.088) normal (1, 0, 0) x (0, 1, 0)
  line L0 (0, 0) -> (152.4, 0) construction
  line L1 (0, -18.288) -> (0, 0) construction
  line L2 (0, 0) -> (2.2451, -2.2451) construction
  circle A0 centre (2.2451, -2.2451) radius 3.175
  dimension "d226" = 3.175
  constraint coincident L0.start L1.end
  constraint coincident L0.start A0
  measures "d226" distance of L0.start L2.end
sweep "Sweep3'" cut kept parallel profiles "Sketch25" along 1 edges at (-9.144, -304.8, 323.088) section 1 on bodies 3 bodies 3 in component "RightSide"
ref_plane "WorkPlane12" through (-18.288, -152.4, 304.8) normal (1, 0, 0) x (0, 1, 0)
sketch "Sketch26" plane through (-18.288, -152.4, 304.8) normal (1, 0, 0) x (0, 1, 0)
  line L0 (0, 18.288) -> (0, 0) construction
  line L1 (0, 0) -> (-152.4, 0) construction
  line L2 (0, 0) -> (-2.2451, 2.2451) construction
  circle A0 centre (-2.2451, 2.2451) radius 3.175
  dimension "d234" = 3.175
  constraint coincident L0.end L1.start
  constraint coincident L0.end A0
  measures "d234" distance of L0.end L2.end
sweep "Sweep4'" cut kept parallel profiles "Sketch26" along 1 edges at (-9.144, -152.4, 304.8) section 1 on bodies 3 bodies 3 in component "RightSide"
ref_plane "WorkPlane13" through (-18.288, -304.8, 304.8) normal (1, 0, 0) x (0, 1, 0)
sketch "Sketch27" plane through (-18.288, -304.8, 304.8) normal (1, 0, 0) x (0, 1, 0)
  line L0 (0, 0) -> (0, 13.7979) construction
  line L1 (147.9099, 0) -> (0, 0) construction
  line L2 (0, 0) -> (2.2451, 2.2451) construction
  circle A0 centre (2.2451, 2.2451) radius 3.175
  dimension "d242" = 3.175
  constraint coincident L0.start L1.end
  constraint coincident L0.start A0
  measures "d242" distance of L0.start L2.end
sweep "Sweep5'" cut kept parallel profiles "Sketch27" along 1 edges at (-9.144, -304.8, 304.8) section 1 on bodies 3 bodies 3 in component "RightSide"
ref_plane "WorkPlane14" through (-18.288, -152.4, 323.088) normal (1, 0, 0) x (0, 1, 0)
sketch "Sketch28" plane through (-18.288, -152.4, 323.088) normal (1, 0, 0) x (0, 1, 0)
  line L0 (0, 0) -> (0, -13.7979) construction
  line L1 (-147.9099, 0) -> (0, 0) construction
  line L2 (0, 0) -> (-2.2451, -2.2451) construction
  circle A0 centre (-2.2451, -2.2451) radius 3.175
  dimension "d250" = 3.175
  constraint coincident L0.start L1.end
  constraint coincident L0.start A0
  measures "d250" distance of L0.start L2.end
sweep "Sweep6'" cut kept parallel profiles "Sketch28" along 1 edges at (-9.144, -152.4, 323.088) section 1 on bodies 3 bodies 3 in component "RightSide"
ref_plane "WorkPlane15" through (0, -304.8, 1364.488) normal (-1, 0, 0) x (0, -1, 0)
sketch "Sketch29" plane through (0, -304.8, 1364.488) normal (-1, 0, 0) x (0, -1, 0)
  line L0 (0, 0) -> (152.4, 0) construction
  line L1 (0, 18.288) -> (0, 0) construction
  line L2 (0, 0) -> (2.2451, 2.2451) construction
  circle A0 centre (2.2451, 2.2451) radius 3.175
  dimension "d258" = 3.175
  constraint coincident L0.start L1.end
  constraint coincident L0.start A0
  measures "d258" distance of L0.start L2.end
sweep "Sweep7'" cut kept parallel profiles "Sketch29" along 1 edges at (-9.144, -304.8, 1364.488) section 1 on bodies 3 bodies 3 in component "RightSide"
ref_plane "WorkPlane16" through (-18.288, -152.4, 1364.488) normal (1, 0, 0) x (0, 1, 0)
sketch "Sketch30" plane through (-18.288, -152.4, 1364.488) normal (1, 0, 0) x (0, 1, 0)
  line L0 (152.4, 0) -> (0, 0) construction
  line L1 (0, 18.288) -> (0, 0) construction
  line L2 (0, 0) -> (2.2451, 2.2451) construction
  circle A0 centre (2.2451, 2.2451) radius 3.175
  dimension "d266" = 3.175
  constraint coincident L0.end L1.end
  constraint coincident L0.end A0
  measures "d266" distance of L0.end L2.end
sweep "Sweep8'" cut kept parallel profiles "Sketch30" along 1 edges at (-9.144, -152.4, 1364.488) section 1 on bodies 3 bodies 3 in component "RightSide"
ref_plane "WorkPlane17" through (-18.288, -18.288, 1262.888) normal (1, 0, 0) x (0, 1, 0)
sketch "Sketch31" plane through (-18.288, -18.288, 1262.888) normal (1, 0, 0) x (0, 1, 0)
  line L0 (0, 0) -> (18.288, 0) construction
  line L1 (0, 50.8) -> (0, 0) construction
  line L2 (0, 0) -> (2.2451, 2.2451) construction
  circle A0 centre (2.2451, 2.2451) radius 3.175
  dimension "d274" = 3.175
  constraint coincident L0.start L1.end
  constraint coincident L0.start A0
  measures "d274" distance of L0.start L2.end
sweep "Sweep9" cut kept parallel profiles "Sketch31" along 1 edges at (-9.144, -18.288, 1262.888) section 1 on bodies 3 bodies 3 in component "RightSide"
ref_plane "WorkPlane18" through (0, -18.288, 1313.688) normal (-1, 0, 0) x (0, -1, 0)
sketch "Sketch32" plane through (0, -18.288, 1313.688) normal (-1, 0, 0) x (0, -1, 0)
  line L0 (0, 0) -> (-18.288, 0) construction
  line L1 (0, -46.3099) -> (0, 0) construction
  line L2 (0, 0) -> (-2.2451, -2.2451) construction
  circle A0 centre (-2.2451, -2.2451) radius 3.175
  dimension "d282" = 3.175
  constraint coincident L0.start L1.end
  constraint coincident L0.start A0
  measures "d282" distance of L0.start L2.end
sweep "Sweep10" cut kept parallel profiles "Sketch32" along 1 edges at (-9.144, -18.288, 1313.688) section 1 on bodies 3 bodies 3 in component "RightSide"
ref_plane "WorkPlane19" through (471.551, -152.4, 0) normal (-1, 0, 0) x (0, -1, 0)
sketch "Sketch33" plane through (471.551, -152.4, 0) normal (-1, 0, 0) x (0, -1, 0)
  line L0 (-152.4, 0) -> (0, 0) construction
  line L1 (0, -18.288) -> (0, 0) construction
  line L2 (0, 0) -> (-2.2451, -2.2451) construction
  circle A0 centre (-2.2451, -2.2451) radius 3.175
  dimension "d290" = 3.175
  constraint coincident L0.end L1.end
  constraint coincident L0.end A0
  measures "d290" distance of L0.end L2.end
sweep "Sweep1''" cut kept parallel profiles "Sketch33" along 1 edges at (462.407, -152.4, 0) section 1 on bodies 4 bodies 4 in component "LeftSide"
ref_plane "WorkPlane20" through (453.263, -304.8, 0) normal (1, 0, 0) x (0, 1, 0)